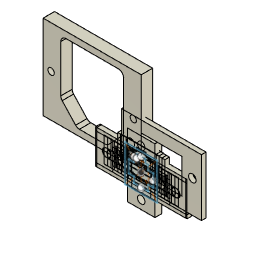
Panel Mount Profiles (Autodesk Fusion 360 design; units mm, degrees)
Autodesk Fusion 360 part; units mm, degrees
(part 1 of 2)
sketch "MF3 1R 2P" plane through (0, 0, 0) normal (0, 1, 0) x (1, 0, 0) in component "Molex Micro Fit 3"
  line L0 (5.75, 1.575) -> (-5.75, 1.575) construction
  line L1 (-5.75, 1.575) -> (-5.75, -1.575)
  line L2 (-5.75, -1.575) -> (5.75, -1.575) construction
  line L3 (5.75, -1.575) -> (5.75, 1.575)
  line L4 (5.75, 1.575) -> (-5.75, -1.575) construction
  line L5 (-5.75, 1.575) -> (5.75, -1.575) construction
  line L6 (3.575, 2.075) -> (-3.575, 2.075)
  line L7 (-3.575, 2.075) -> (-3.575, -2.075) construction
  line L8 (-3.575, -2.075) -> (3.575, -2.075) construction
  line L9 (3.575, -2.075) -> (3.575, 2.075) construction
  line L10 (3.575, 2.075) -> (-3.575, -2.075) construction
  line L11 (-3.575, 2.075) -> (3.575, -2.075) construction
  line L12 (0, -2.075) -> (0, -3.275) construction
  line L13 (1.45, -3.275) -> (-1.45, -3.275)
  line L14 (-1.45, -3.275) -> (-1.45, -2.075)
  line L15 (-1.45, -2.075) -> (1.45, -2.075) construction
  line L16 (1.45, -2.075) -> (1.45, -3.275)
  line L17 (1.45, -3.275) -> (-1.45, -2.075) construction
  line L18 (-1.45, -3.275) -> (1.45, -2.075) construction
  line L19 (3.575, 1.575) -> (3.575, 2.075)
  line L20 (3.575, 1.575) -> (5.75, 1.575)
  line L21 (-5.75, 1.575) -> (-3.575, 1.575)
  line L22 (-3.575, 1.575) -> (-3.575, 2.075)
  line L23 (-5.75, -1.575) -> (-3.575, -1.575)
  line L24 (-3.575, -1.575) -> (-3.575, -2.075)
  line L25 (-3.575, -2.075) -> (-1.45, -2.075)
  line L26 (1.45, -2.075) -> (3.575, -2.075)
  line L27 (3.575, -2.075) -> (3.575, -1.575)
  line L28 (3.575, -1.575) -> (5.75, -1.575)
  line L29 (0, -3.275) -> (0, 2.075) construction
  line L30 (7.25, 3.4) -> (-7.25, 3.4)
  line L31 (-7.25, 3.4) -> (-7.25, -4.6)
  line L32 (-7.25, -4.6) -> (7.25, -4.6)
  line L33 (7.25, -4.6) -> (7.25, 3.4)
  line L34 (7.25, 3.4) -> (-7.25, -4.6) construction
  line L35 (-7.25, 3.4) -> (7.25, -4.6) construction
  point P0 (0, -2.675)
  point P1 (0, -0.6)
  dimension "d223" = 11.5
  dimension "d224" = 3.15
  dimension "d225" = 7.15
  dimension "d226" = 4.15
  dimension "d227" = 1.2
  dimension "d228" = 2.9
  dimension "d229" = 14.5
  dimension "d230" = 5.35
  dimension "d231" = 8
  constraint horizontal L0
  constraint perpendicular L0 L1
  constraint parallel L0 L2
  constraint parallel L1 L3
  constraint coincident L4 origin
  constraint coincident L5 origin
  constraint horizontal L6
  constraint perpendicular L6 L7
  constraint parallel L6 L8
  constraint parallel L7 L9
  constraint coincident L10 origin
  constraint coincident L11 origin
  constraint midpoint L8 L12.start
  constraint perpendicular L8 L12
  constraint horizontal L13
  constraint perpendicular L13 L14
  constraint parallel L13 L15
  constraint parallel L14 L16
  constraint coincident L17 P0
  constraint coincident L18 P0
  constraint midpoint L12 P0
  constraint coincident L0 L19.start
  constraint coincident L9 L19.start
  constraint perpendicular L3 L20
  constraint coincident L0 L21.end
  constraint coincident L7 L21.end
  constraint coincident L2 L23.end
  constraint coincident L7 L23.end
  constraint perpendicular L14 L25
  constraint coincident L2 L27.end
  constraint coincident L9 L27.end
  constraint midpoint L6 L29.end
  constraint horizontal L30
  constraint perpendicular L30 L31
  constraint parallel L30 L32
  constraint parallel L31 L33
  constraint coincident L34 P1
  constraint coincident L35 P1
  constraint midpoint L29 P1
  measures "d223" distance of L1.end L2.end
  measures "d224" distance of L0.end L1.end
  measures "d225" distance of L7.end L8.end
  measures "d226" distance of L6.end L7.end
  measures "d227" distance of L12.start L12.end
  measures "d228" distance of L14.end L15.end
  measures "d229" distance of L31.end L32.end
  measures "d230" distance of L6 L13
  measures "d231" distance of L30.end L31.end
sketch "MF3 2R 2P" plane through (0, 0, 0) normal (0, 1, 0) x (1, 0, 0) in component "Molex Micro Fit 3"
  line L0 (-5.6125, 4.8465) -> (5.8875, 4.8465)
  line L1 (5.8875, 4.8465) -> (5.8875, -6.1535)
  line L2 (5.8875, -6.1535) -> (-5.6125, -6.1535)
  line L3 (-5.6125, -6.1535) -> (-5.6125, 4.8465)
  line L4 (-5.6125, 4.8465) -> (5.8875, -6.1535) construction
  line L5 (5.8875, 4.8465) -> (-5.6125, -6.1535) construction
  line L6 (4.25, 1.875) -> (-4.25, 1.875) construction
  line L7 (-4.25, 1.875) -> (-4.25, -1.875)
  line L8 (-4.25, -1.875) -> (4.25, -1.875) construction
  line L9 (4.25, -1.875) -> (4.25, 1.875)
  line L10 (4.25, 1.875) -> (-4.25, -1.875) construction
  line L11 (-4.25, 1.875) -> (4.25, -1.875) construction
  line L12 (2.075, 3.575) -> (-2.075, 3.575)
  line L13 (-2.075, 3.575) -> (-2.075, -3.575) construction
  line L14 (-2.075, -3.575) -> (2.075, -3.575) construction
  line L15 (2.075, -3.575) -> (2.075, 3.575) construction
  line L16 (2.075, 3.575) -> (-2.075, -3.575) construction
  line L17 (-2.075, 3.575) -> (2.075, -3.575) construction
  line L18 (0, -3.575) -> (0, -4.775) construction
  line L19 (0.85, -4.775) -> (-0.85, -4.775)
  line L20 (-0.85, -4.775) -> (-0.85, -3.575)
  line L21 (-0.85, -3.575) -> (0.85, -3.575) construction
  line L22 (0.85, -3.575) -> (0.85, -4.775)
  line L23 (0.85, -4.775) -> (-0.85, -3.575) construction
  line L24 (-0.85, -4.775) -> (0.85, -3.575) construction
  line L25 (0.1375, -6.1535) -> (0.1375, 4.8465) construction
  line L26 (0.85, -3.575) -> (2.075, -3.575)
  line L27 (2.075, -1.875) -> (4.25, -1.875)
  line L28 (2.075, -1.875) -> (2.075, -3.575)
  line L29 (4.25, 1.875) -> (2.075, 1.875)
  line L30 (2.075, 1.875) -> (2.075, 3.575)
  line L31 (-2.075, 3.575) -> (-2.075, 1.875)
  line L32 (-2.075, 1.875) -> (-4.25, 1.875)
  line L33 (-4.25, -1.875) -> (-2.075, -1.875)
  line L34 (-2.075, -1.875) -> (-2.075, -3.575)
  line L35 (-2.075, -3.575) -> (-0.85, -3.575)
  point P0 (0.1375, -0.6535)
  point P1 (0, -4.175)
  dimension "d105" = 11.5
  dimension "d106" = 11
  dimension "d162" = 8.5
  dimension "d163" = 3.75
  dimension "d164" = 4.15
  dimension "d165" = 7.15
  dimension "d166" = 1.2
  dimension "d167" = 1.7
  constraint horizontal L0
  constraint perpendicular L0 L1
  constraint parallel L0 L2
  constraint parallel L1 L3
  constraint coincident L4 P0
  constraint coincident L5 P0
  constraint horizontal L6
  constraint perpendicular L6 L7
  constraint parallel L6 L8
  constraint parallel L7 L9
  constraint coincident L10 origin
  constraint coincident L11 origin
  constraint horizontal L12
  constraint perpendicular L12 L13
  constraint parallel L12 L14
  constraint parallel L13 L15
  constraint coincident L16 origin
  constraint coincident L17 origin
  constraint midpoint L14 L18.start
  constraint perpendicular L14 L18
  constraint horizontal L19
  constraint perpendicular L19 L20
  constraint parallel L19 L21
  constraint parallel L20 L22
  constraint coincident L23 P1
  constraint coincident L24 P1
  constraint midpoint L18 P1
  constraint coincident L18.end L19
  constraint midpoint L2 L25.start
  constraint midpoint L0 L25.end
  constraint coincident L15 L27.start
  constraint coincident L8 L27.start
  constraint coincident L6 L29.end
  constraint coincident L15 L29.end
  constraint coincident L13 L31.end
  constraint coincident L6 L31.end
  constraint coincident L13 L33.end
  constraint coincident L8 L33.end
  measures "d105" distance of L1.end L2.end
  measures "d106" distance of L0.end L1.end
  measures "d162" distance of L7.end L8.end
  measures "d163" distance of L6.end L7.end
  measures "d164" distance of L13.end L14.end
  measures "d165" distance of L12.end L13.end
  measures "d166" distance of L18.start L18.end
  measures "d167" distance of L20.end L21.end
sketch "MF3 1R 3P" plane through (0, 0, 0) normal (0, 1, 0) x (1, 0, 0) in component "Molex Micro Fit 3"
  line L0 (0.0006, -3.28) -> (0.0006, 2.09) construction
  line L1 (5.0756, -2.06) -> (5.0756, 2.09) construction
  line L2 (5.0756, 2.09) -> (-5.0744, 2.09)
  line L3 (-5.0744, 2.09) -> (-5.0744, -2.08) construction
  line L4 (-5.0744, -2.08) -> (-1.4494, -2.08)
  line L5 (-1.4494, -3.28) -> (-1.4494, -2.08)
  line L6 (1.4506, -3.28) -> (-1.4494, -3.28)
  line L7 (1.4506, -2.06) -> (1.4506, -3.28)
  line L8 (1.4506, -2.06) -> (5.0756, -2.06)
  line L9 (7.25, -1.575) -> (-7.25, -1.575) construction
  line L10 (-7.25, -1.575) -> (-7.25, 1.575)
  line L11 (-7.25, 1.575) -> (7.25, 1.575) construction
  line L12 (7.25, 1.575) -> (7.25, -1.575)
  line L13 (7.25, -1.575) -> (-7.25, 1.575) construction
  line L14 (-7.25, -1.575) -> (7.25, 1.575) construction
  line L15 (-5.0744, -2.08) -> (-5.0744, -1.575)
  line L16 (-5.0744, -1.575) -> (-7.25, -1.575)
  line L17 (-7.25, 1.575) -> (-5.0744, 1.575)
  line L18 (-5.0744, 1.575) -> (-5.0744, 2.09)
  line L19 (5.0756, 2.09) -> (5.0756, 1.5652)
  line L20 (5.0756, 1.5652) -> (7.25, 1.575)
  line L21 (7.25, -1.575) -> (5.0756, -1.575)
  line L22 (5.0756, -1.575) -> (5.0756, -2.06)
  line L23 (8.7506, 3.405) -> (-8.7494, 3.405)
  line L24 (-8.7494, 3.405) -> (-8.7494, -4.595)
  line L25 (-8.7494, -4.595) -> (8.7506, -4.595)
  line L26 (8.7506, -4.595) -> (8.7506, 3.405)
  line L27 (8.7506, 3.405) -> (-8.7494, -4.595) construction
  line L28 (-8.7494, 3.405) -> (8.7506, -4.595) construction
  point P0 (0.0006, -0.595)
  dimension "d96" = 14.5
  dimension "d97" = 3.15
  dimension "d98" = 17.5
  dimension "d99" = 8
  dimension "d129" = 1.2
  dimension "d130" = 2.9
  dimension "d131" = 4.15
  dimension "d132" = 10.15
  dimension "d133" = 5.37
  constraint horizontal L9
  constraint perpendicular L9 L10
  constraint parallel L9 L11
  constraint parallel L10 L12
  constraint coincident L13 origin
  constraint coincident L14 origin
  constraint coincident L9 L15.end
  constraint coincident L3 L15.end
  constraint coincident L11 L17.end
  constraint coincident L3 L17.end
  constraint coincident L1 L19.end
  constraint coincident L9 L21.end
  constraint coincident L1 L21.end
  constraint horizontal L23
  constraint perpendicular L23 L24
  constraint parallel L23 L25
  constraint parallel L24 L26
  constraint coincident L27 P0
  constraint coincident L28 P0
  constraint midpoint L0 P0
  constraint midpoint L0.start L6
  constraint midpoint L0.end L2
  constraint horizontal L8
  constraint horizontal L4
  constraint horizontal L2
  constraint vertical L3
  constraint vertical L1
  constraint vertical L5
  constraint vertical L7
  constraint symmetric L0 L24 L26
  measures "d96" distance of L10.end L11.end
  measures "d97" distance of L9.end L10.end
  measures "d98" distance of L24.end L25.end
  measures "d99" distance of L23.end L24.end
  measures "d129" distance of L4.end L5.start
  measures "d130" distance of L5.start L6.start
  measures "d131" distance of L1.start L1.end
  measures "d132" distance of L1.end L2.end
  measures "d133" distance of L2 L6
sketch "MF3 1R 4P" plane through (0, 0, 0) normal (0, 1, 0) x (1, 0, 0) in component "Molex Micro Fit 3"
  line L0 (6.575, 2.075) -> (-6.575, 2.075)
  line L1 (6.575, 2.075) -> (-6.575, -2.075) construction
  line L2 (-6.575, 2.075) -> (6.575, -2.075) construction
  line L3 (0, -2.075) -> (0, -3.275) construction
  line L4 (1.45, -3.275) -> (-1.45, -3.275)
  line L5 (-1.45, -3.275) -> (-1.45, -2.075)
  line L6 (-1.45, -2.075) -> (1.45, -2.075) construction
  line L7 (1.45, -2.075) -> (1.45, -3.275)
  line L8 (1.45, -3.275) -> (-1.45, -2.075) construction
  line L9 (-1.45, -3.275) -> (1.45, -2.075) construction
  line L10 (-6.575, -2.075) -> (-1.45, -2.075)
  line L11 (0, -2.075) -> (6.575, -2.075)
  line L12 (8.75, 1.575) -> (-8.75, 1.575)
  line L13 (-8.75, 1.575) -> (-8.75, -1.575)
  line L14 (-8.75, -1.575) -> (8.75, -1.575)
  line L15 (8.75, -1.575) -> (8.75, 1.575)
  line L16 (8.75, 1.575) -> (-8.75, -1.575) construction
  line L17 (-8.75, 1.575) -> (8.75, -1.575) construction
  line L18 (6.575, -2.075) -> (6.575, -1.575)
  line L19 (6.575, 1.575) -> (6.575, 2.075)
  line L20 (-6.575, 2.075) -> (-6.575, 1.575)
  line L21 (-6.575, -1.575) -> (-6.575, -2.075)
  line L22 (0, -3.275) -> (0, 2.075) construction
  line L23 (10.75, 3.4) -> (-10.75, 3.4)
  line L24 (-10.75, 3.4) -> (-10.75, -4.6)
  line L25 (-10.75, -4.6) -> (10.75, -4.6)
  line L26 (10.75, -4.6) -> (10.75, 3.4)
  line L27 (10.75, 3.4) -> (-10.75, -4.6) construction
  line L28 (-10.75, 3.4) -> (10.75, -4.6) construction
  point P0 (0, -2.675)
  point P1 (0, -0.6)
  dimension "d120" = 13.15
  dimension "d121" = 4.15
  dimension "d122" = 1.2
  dimension "d123" = 2.9
  dimension "d124" = 17.5
  dimension "d125" = 3.15
  dimension "d126" = 5.35
  dimension "d127" = 8
  dimension "d128" = 21.5
  constraint horizontal L0
  constraint perpendicular L0 L20
  constraint parallel L0 L10
  constraint parallel L18 L20
  constraint coincident L1 origin
  constraint coincident L2 origin
  constraint perpendicular L3 L10
  constraint horizontal L4
  constraint perpendicular L4 L5
  constraint parallel L4 L6
  constraint parallel L5 L7
  constraint coincident L8 P0
  constraint coincident L9 P0
  constraint midpoint L3 P0
  constraint collinear L10 L11
  constraint coincident L3.start L10
  constraint horizontal L12
  constraint perpendicular L12 L13
  constraint parallel L12 L14
  constraint parallel L13 L15
  constraint coincident L16 origin
  constraint coincident L17 origin
  constraint collinear L18 L19
  constraint collinear L20 L21
  constraint coincident L14 L21.start
  constraint coincident L12 L20.end
  constraint coincident L12 L19.start
  constraint coincident L14 L18.end
  constraint midpoint L0 L22.end
  constraint perpendicular L0 L22
  constraint horizontal L23
  constraint perpendicular L23 L24
  constraint parallel L23 L25
  constraint parallel L24 L26
  constraint coincident L27 P1
  constraint coincident L28 P1
  constraint midpoint L22 P1
  measures "d120" distance of L1.end L2.end
  measures "d121" distance of L0.end L1.end
  measures "d122" distance of L3.start L3.end
  measures "d123" distance of L5.end L6.end
  measures "d124" distance of L13.end L14.end
  measures "d125" distance of L12.end L13.end
  measures "d126" distance of L0 L4
  measures "d127" distance of L23.end L24.end
  measures "d128" distance of L23.start L23.end
sketch "MF3 1R 5P" plane through (0, 0, 0) normal (0, 1, 0) x (1, 0, 0) in component "Molex Micro Fit 3"
  line L0 (10.25, 1.575) -> (-10.25, 1.575)
  line L1 (-10.25, 1.575) -> (-10.25, -1.575)
  line L2 (-10.25, -1.575) -> (10.25, -1.575)
  line L3 (10.25, -1.575) -> (10.25, 1.575)
  line L4 (10.25, 1.575) -> (-10.25, -1.575) construction
  line L5 (-10.25, 1.575) -> (10.25, -1.575) construction
  line L6 (8.075, 2.075) -> (-8.075, 2.075)
  line L7 (-8.075, 2.075) -> (-8.075, -2.075)
  line L8 (-8.075, -2.075) -> (8.075, -2.075)
  line L9 (8.075, -2.075) -> (8.075, 2.075)
  line L10 (8.075, 2.075) -> (-8.075, -2.075) construction
  line L11 (-8.075, 2.075) -> (8.075, -2.075) construction
  line L12 (0, -2.075) -> (0, -3.275) construction
  line L13 (1.45, -2.075) -> (-1.45, -2.075)
  line L14 (-1.45, -2.075) -> (-1.45, -3.275)
  line L15 (-1.45, -3.275) -> (1.45, -3.275)
  line L16 (1.45, -3.275) -> (1.45, -2.075)
  line L17 (1.45, -2.075) -> (-1.45, -3.275) construction
  line L18 (-1.45, -2.075) -> (1.45, -3.275) construction
  line L19 (0, -3.275) -> (0, 2.075) construction
  line L20 (11.25, 3.4) -> (-11.25, 3.4)
  line L21 (-11.25, 3.4) -> (-11.25, -4.6)
  line L22 (-11.25, -4.6) -> (11.25, -4.6)
  line L23 (11.25, -4.6) -> (11.25, 3.4)
  line L24 (11.25, 3.4) -> (-11.25, -4.6) construction
  line L25 (-11.25, 3.4) -> (11.25, -4.6) construction
  point P0 (0, -2.675)
  point P1 (0, -0.6)
  dimension "d134" = 20.5
  dimension "d135" = 3.15
  dimension "d136" = 16.15
  dimension "d137" = 4.15
  dimension "d138" = 1.2
  dimension "d139" = 2.9
  dimension "d140" = 1.2
  dimension "d141" = 5.35
  dimension "d142" = 22.5
  dimension "d143" = 8
  constraint horizontal L0
  constraint perpendicular L0 L1
  constraint parallel L0 L2
  constraint parallel L1 L3
  constraint coincident L4 origin
  constraint coincident L5 origin
  constraint horizontal L6
  constraint perpendicular L6 L7
  constraint parallel L6 L8
  constraint parallel L7 L9
  constraint coincident L10 origin
  constraint coincident L11 origin
  constraint midpoint L8 L12.start
  constraint perpendicular L8 L12
  constraint horizontal L13
  constraint perpendicular L13 L14
  constraint parallel L13 L15
  constraint parallel L14 L16
  constraint coincident L17 P0
  constraint coincident L18 P0
  constraint midpoint L12 P0
  constraint midpoint L6 L19.end
  constraint horizontal L20
  constraint perpendicular L20 L21
  constraint parallel L20 L22
  constraint parallel L21 L23
  constraint coincident L24 P1
  constraint coincident L25 P1
  constraint midpoint L19 P1
  measures "d134" distance of L1.end L2.end
  measures "d135" distance of L0.end L1.end
  measures "d136" distance of L7.end L8.end
  measures "d137" distance of L6.end L7.end
  measures "d138" distance of L12.start L12.end
  measures "d139" distance of L14.end L15.end
  measures "d140" distance of L13.end L14.end
  measures "d141" distance of L6 L15
  measures "d142" distance of L21.end L22.end
  measures "d143" distance of L20.end L21.end
sketch "MF3 2R 4P" plane through (0, 0, 0) normal (0, 1, 0) x (1, 0, 0) in component "Molex Micro Fit 3"
  line L0 (3.575, 3.45) -> (-3.575, 3.45)
  line L1 (-3.575, 3.45) -> (-3.575, -3.45) construction
  line L2 (-3.575, -3.45) -> (3.575, -3.45) construction
  line L3 (3.575, -3.45) -> (3.575, 3.45) construction
  line L4 (3.575, 3.45) -> (-3.575, -3.45) construction
  line L5 (-3.575, 3.45) -> (3.575, -3.45) construction
  line L6 (5.75, 1.875) -> (-5.75, 1.875) construction
  line L7 (-5.75, 1.875) -> (-5.75, -1.875)
  line L8 (-5.75, -1.875) -> (5.75, -1.875) construction
  line L9 (5.75, -1.875) -> (5.75, 1.875)
  line L10 (5.75, 1.875) -> (-5.75, -1.875) construction
  line L11 (-5.75, 1.875) -> (5.75, -1.875) construction
  line L12 (0, -3.45) -> (0, -4.85) construction
  line L13 (0.85, -4.85) -> (-0.85, -4.85)
  line L14 (-0.85, -4.85) -> (-0.85, -3.45)
  line L15 (0.85, -3.45) -> (0.85, -4.85)
  line L16 (0.85, -4.85) -> (-0.85, -3.45) construction
  line L17 (-0.85, -4.85) -> (0.85, -3.45) construction
  line L18 (5.75, -1.875) -> (3.575, -1.875)
  line L19 (3.575, -1.875) -> (3.575, -3.45)
  line L20 (3.575, -3.45) -> (0.85, -3.45)
  line L21 (-0.85, -3.45) -> (-3.575, -3.45)
  line L22 (-3.575, -3.45) -> (-3.575, -1.875)
  line L23 (-3.575, -1.875) -> (-5.75, -1.875)
  line L24 (-5.75, 1.875) -> (-3.575, 1.875)
  line L25 (-3.575, 1.875) -> (-3.575, 3.45)
  line L26 (3.575, 3.45) -> (3.575, 1.875)
  line L27 (3.575, 1.875) -> (5.75, 1.875)
  line L28 (0, -4.85) -> (0, 3.45) construction
  line L29 (7.25, 4.8) -> (-7.25, 4.8)
  line L30 (-7.25, 4.8) -> (-7.25, -6.2)
  line L31 (-7.25, -6.2) -> (7.25, -6.2)
  line L32 (7.25, -6.2) -> (7.25, 4.8)
  line L33 (7.25, 4.8) -> (-7.25, -6.2) construction
  line L34 (-7.25, 4.8) -> (7.25, -6.2) construction
  point P0 (0, -4.15)
  point P1 (0, -0.7)
  point P2 (0, -0.7)
  dimension "d176" = 7.15
  dimension "d177" = 6.9
  dimension "d178" = 11.5
  dimension "d179" = 3.75
  dimension "d180" = 1.4
  dimension "d181" = 1.7
  dimension "d184" = 11
  dimension "d185" = 14.5
  constraint horizontal L0
  constraint perpendicular L0 L1
  constraint parallel L0 L2
  constraint parallel L1 L3
  constraint coincident L4 origin
  constraint coincident L5 origin
  constraint horizontal L6
  constraint perpendicular L6 L7
  constraint parallel L6 L8
  constraint parallel L7 L9
  constraint coincident L10 origin
  constraint coincident L11 origin
  constraint midpoint L2 L12.start
  constraint perpendicular L2 L12
  constraint horizontal L13
  constraint perpendicular L13 L14
  constraint parallel L14 L15
  constraint coincident L16 P0
  constraint coincident L17 P0
  constraint midpoint L12 P0
  constraint coincident L12.end L13
  constraint coincident L8 L18.end
  constraint coincident L3 L18.end
  constraint perpendicular L15 L20
  constraint coincident L1 L22.end
  constraint coincident L8 L22.end
  constraint coincident L1 L24.end
  constraint coincident L6 L24.end
  constraint coincident L3 L26.end
  constraint coincident L6 L26.end
  constraint midpoint L0 L28.end
  constraint midpoint L28 P2
  constraint horizontal L29
  constraint perpendicular L29 L30
  constraint parallel L29 L31
  constraint parallel L30 L32
  constraint coincident L33 P2
  constraint coincident L34 P2
  constraint coincident P2 P1
  measures "d176" distance of L1.end L2.end
  measures "d177" distance of L0.end L1.end
  measures "d178" distance of L7.end L8.end
  measures "d179" distance of L6.end L7.end
  measures "d180" distance of L12.start L12.end
  measures "d181" distance of L14.end L15.start
  measures "d184" distance of L29.end L30.end
  measures "d185" distance of L30 L32
sketch "MF3 2R 8P" plane through (0, 0, 0) normal (0, 1, 0) x (1, 0, 0) in component "Molex Micro Fit 3"
  line L0 (6.575, 3.575) -> (-6.575, 3.575)
  line L1 (-6.575, 3.575) -> (-6.575, -3.575) construction
  line L2 (-6.575, -3.575) -> (6.575, -3.575) construction
  line L3 (6.575, -3.575) -> (6.575, 3.575) construction
  line L4 (6.575, 3.575) -> (-6.575, -3.575) construction
  line L5 (-6.575, 3.575) -> (6.575, -3.575) construction
  line L6 (8.75, 1.875) -> (-8.75, 1.875) construction
  line L7 (-8.75, 1.875) -> (-8.75, -1.875)
  line L8 (-8.75, -1.875) -> (8.75, -1.875) construction
  line L9 (8.75, -1.875) -> (8.75, 1.875)
  line L10 (8.75, 1.875) -> (-8.75, -1.875) construction
  line L11 (-8.75, 1.875) -> (8.75, -1.875) construction
  line L12 (0, -3.575) -> (0, -4.975) construction
  line L13 (0.85, -3.575) -> (-0.85, -3.575) construction
  line L14 (-0.85, -3.575) -> (-0.85, -4.975)
  line L15 (-0.85, -4.975) -> (0.85, -4.975)
  line L16 (0.85, -4.975) -> (0.85, -3.575)
  line L17 (0.85, -3.575) -> (-0.85, -4.975) construction
  line L18 (-0.85, -3.575) -> (0.85, -4.975) construction
  line L19 (8.75, -1.875) -> (6.575, -1.875)
  line L20 (6.575, -1.875) -> (6.575, -3.575)
  line L21 (6.575, -3.575) -> (0.85, -3.575)
  line L22 (8.75, 1.875) -> (6.575, 1.875)
  line L23 (6.575, 1.875) -> (6.575, 3.575)
  line L24 (-6.575, 3.575) -> (-6.575, 1.875)
  line L25 (-6.575, 1.875) -> (-8.75, 1.875)
  line L26 (-8.75, -1.875) -> (-6.575, -1.875)
  line L27 (-6.575, -1.875) -> (-6.575, -3.575)
  line L28 (-6.575, -3.575) -> (-0.85, -3.575)
  line L29 (0, -4.975) -> (0, 3.575) construction
  line L30 (10.25, 4.8) -> (-10.25, 4.8)
  line L31 (-10.25, 4.8) -> (-10.25, -6.2)
  line L32 (-10.25, -6.2) -> (10.25, -6.2)
  line L33 (10.25, -6.2) -> (10.25, 4.8)
  line L34 (10.25, 4.8) -> (-10.25, -6.2) construction
  line L35 (-10.25, 4.8) -> (10.25, -6.2) construction
  point P0 (0, -4.275)
  point P1 (0, -0.7)
  dimension "d186" = 13.15
  dimension "d187" = 7.15
  dimension "d188" = 17.5
  dimension "d189" = 3.75
  dimension "d190" = 1.4
  dimension "d191" = 1.7
  dimension "d192" = 20.5
  dimension "d193" = 11
  constraint horizontal L0
  constraint perpendicular L0 L1
  constraint parallel L0 L2
  constraint parallel L1 L3
  constraint coincident L4 origin
  constraint coincident L5 origin
  constraint horizontal L6
  constraint perpendicular L6 L7
  constraint parallel L6 L8
  constraint parallel L7 L9
  constraint coincident L10 origin
  constraint coincident L11 origin
  constraint midpoint L2 L12.start
  constraint perpendicular L2 L12
  constraint horizontal L13
  constraint perpendicular L13 L14
  constraint parallel L13 L15
  constraint parallel L14 L16
  constraint coincident L17 P0
  constraint coincident L18 P0
  constraint midpoint L12 P0
  constraint coincident L12.end L15
  constraint coincident L8 L19.end
  constraint coincident L3 L19.end
  constraint coincident L6 L22.end
  constraint coincident L3 L22.end
  constraint coincident L6 L24.end
  constraint coincident L1 L24.end
  constraint coincident L8 L26.end
  constraint coincident L1 L26.end
  constraint midpoint L0 L29.end
  constraint horizontal L30
  constraint perpendicular L30 L31
  constraint parallel L30 L32
  constraint parallel L31 L33
  constraint coincident L34 P1
  constraint coincident L35 P1
  constraint midpoint L29 P1
  measures "d186" distance of L1.end L2.end
  measures "d187" distance of L0.end L1.end
  measures "d188" distance of L7.end L8.end
  measures "d189" distance of L6.end L7.end
  measures "d190" distance of L12.start L12.end
  measures "d191" distance of L14.end L15.end
  measures "d192" distance of L31.end L32.end
  measures "d193" distance of L30.end L31.end
sketch "MF3 2R 6P" plane through (0, 0, 0) normal (0, 1, 0) x (1, 0, 0) in component "Molex Micro Fit 3"
  line L0 (5.075, 3.575) -> (-5.075, 3.575)
  line L1 (-5.075, 3.575) -> (-5.075, -3.575) construction
  line L2 (-5.075, -3.575) -> (5.075, -3.575) construction
  line L3 (5.075, -3.575) -> (5.075, 3.575) construction
  line L4 (5.075, 3.575) -> (-5.075, -3.575) construction
  line L5 (-5.075, 3.575) -> (5.075, -3.575) construction
  line L6 (7.25, 1.875) -> (-7.25, 1.875) construction
  line L7 (-7.25, 1.875) -> (-7.25, -1.875)
  line L8 (-7.25, -1.875) -> (7.25, -1.875) construction
  line L9 (7.25, -1.875) -> (7.25, 1.875)
  line L10 (7.25, 1.875) -> (-7.25, -1.875) construction
  line L11 (-7.25, 1.875) -> (7.25, -1.875) construction
  line L12 (0, -3.575) -> (0, -4.975) construction
  line L13 (0.85, -4.975) -> (-0.85, -4.975)
  line L14 (-0.85, -4.975) -> (-0.85, -3.575)
  line L15 (-0.85, -3.575) -> (0.85, -3.575) construction
  line L16 (0.85, -3.575) -> (0.85, -4.975)
  line L17 (0.85, -4.975) -> (-0.85, -3.575) construction
  line L18 (-0.85, -4.975) -> (0.85, -3.575) construction
  line L19 (-0.85, -3.575) -> (-5.075, -3.575)
  line L20 (-5.075, -3.575) -> (-5.075, -1.875)
  line L21 (-5.075, -1.875) -> (-7.25, -1.875)
  line L22 (-7.25, 1.875) -> (-5.075, 1.875)
  line L23 (-5.075, 1.875) -> (-5.075, 3.575)
  line L24 (5.075, 1.875) -> (5.075, 3.575)
  line L25 (5.075, 1.875) -> (7.25, 1.875)
  line L26 (5.075, -3.575) -> (5.075, -1.875)
  line L27 (5.075, -1.875) -> (7.25, -1.875)
  line L28 (0.85, -3.575) -> (5.075, -3.575)
  line L29 (0, -4.975) -> (0, 3.575) construction
  line L30 (8.75, -6.2) -> (-8.75, -6.2)
  line L31 (-8.75, -6.2) -> (-8.75, 4.8)
  line L32 (-8.75, 4.8) -> (8.75, 4.8)
  line L33 (8.75, 4.8) -> (8.75, -6.2)
  line L34 (8.75, -6.2) -> (-8.75, 4.8) construction
  line L35 (-8.75, -6.2) -> (8.75, 4.8) construction
  point P0 (0, -4.275)
  point P1 (0, -0.7)
  dimension "d305" = 10.15
  dimension "d306" = 7.15
  dimension "d307" = 14.5
  dimension "d308" = 3.75
  dimension "d309" = 1.4
  dimension "d310" = 1.7
  dimension "d312" = 17.5
  dimension "d313" = 11
  constraint horizontal L0
  constraint perpendicular L0 L1
  constraint parallel L0 L2
  constraint parallel L1 L3
  constraint coincident L4 origin
  constraint coincident L5 origin
  constraint horizontal L6
  constraint perpendicular L6 L7
  constraint parallel L6 L8
  constraint parallel L7 L9
  constraint coincident L10 origin
  constraint coincident L11 origin
  constraint midpoint L2 L12.start
  constraint perpendicular L2 L12
  constraint horizontal L13
  constraint perpendicular L13 L14
  constraint parallel L13 L15
  constraint parallel L14 L16
  constraint coincident L17 P0
  constraint coincident L18 P0
  constraint midpoint L12 P0
  constraint perpendicular L1 L19
  constraint coincident L8 L20.end
  constraint coincident L1 L20.end
  constraint coincident L6 L22.end
  constraint coincident L1 L22.end
  constraint coincident L6 L24.start
  constraint coincident L3 L24.start
  constraint coincident L3 L26.end
  constraint coincident L8 L26.end
  constraint midpoint L0 L29.end
  constraint horizontal L30
  constraint perpendicular L30 L31
  constraint parallel L30 L32
  constraint parallel L31 L33
  constraint coincident L34 P1
  constraint coincident L35 P1
  constraint midpoint L29 P1
  measures "d305" distance of L1.end L2.end
  measures "d306" distance of L0.end L1.end
  measures "d307" distance of L7.end L8.end
  measures "d308" distance of L6.end L7.end
  measures "d309" distance of L12.start L12.end
  measures "d310" distance of L14.end L15.end
  measures "d312" distance of L30.start L30.end
  measures "d313" distance of L30.end L31.end
sketch "MF3 2R 10P" plane through (0, 0, 0) normal (0, 1, 0) x (1, 0, 0) in component "Molex Micro Fit 3"
  line L0 (11.75, -6.2) -> (-11.75, -6.2)
  line L1 (-8.075, -3.575) -> (8.075, -3.575) construction
  line L2 (0.85, -4.975) -> (-0.85, -4.975)
  line L3 (11.75, 4.8) -> (11.75, -6.2)
  line L4 (-11.75, 4.8) -> (11.75, 4.8)
  line L5 (-10.25, 1.875) -> (-8.075, 1.875)
  line L6 (0, -4.975) -> (0, 3.575) construction
  line L7 (10.25, 1.875) -> (-10.25, 1.875) construction
  line L8 (0, -3.575) -> (0, -4.975) construction
  line L9 (0.85, -3.575) -> (8.075, -3.575)
  line L10 (0.85, -4.975) -> (-0.85, -3.575) construction
  line L11 (8.075, 1.875) -> (8.075, 3.575)
  line L12 (8.075, 1.875) -> (10.25, 1.875)
  line L13 (0.85, -3.575) -> (0.85, -4.975)
  line L14 (-10.25, -1.875) -> (10.25, -1.875) construction
  line L15 (-8.075, -3.575) -> (-8.075, -1.875)
  line L16 (10.25, -1.875) -> (10.25, 1.875)
  line L17 (-8.075, 3.575) -> (-8.075, -3.575) construction
  line L18 (11.75, -6.2) -> (-11.75, 4.8) construction
  line L19 (-0.85, -3.575) -> (-8.075, -3.575)
  line L20 (-0.85, -4.975) -> (-0.85, -3.575)
  line L21 (-0.85, -4.975) -> (0.85, -3.575) construction
  line L22 (8.075, -1.875) -> (10.25, -1.875)
  line L23 (8.075, -3.575) -> (8.075, 3.575) construction
  line L24 (-11.75, -6.2) -> (11.75, 4.8) construction
  line L25 (-10.25, 1.875) -> (10.25, -1.875) construction
  line L26 (10.25, 1.875) -> (-10.25, -1.875) construction
  line L27 (8.075, 3.575) -> (-8.075, -3.575) construction
  line L28 (8.075, 3.575) -> (-8.075, 3.575)
  line L29 (-10.25, 1.875) -> (-10.25, -1.875)
  line L30 (-0.85, -3.575) -> (0.85, -3.575) construction
  line L31 (-8.075, 3.575) -> (8.075, -3.575) construction
  line L32 (-11.75, -6.2) -> (-11.75, 4.8)
  line L33 (-8.075, -1.875) -> (-10.25, -1.875)
  line L34 (-8.075, 1.875) -> (-8.075, 3.575)
  line L35 (8.075, -3.575) -> (8.075, -1.875)
  point P0 (0, -0.7)
  point P1 (0, -4.275)
  dimension "d314" = 16.15
  dimension "d315" = 7.15
  dimension "d316" = 20.5
  dimension "d317" = 3.75
  dimension "d318" = 1.4
  dimension "d319" = 1.7
  dimension "d320" = 23.5
  dimension "d321" = 11
  constraint horizontal L28
  constraint perpendicular L17 L28
  constraint parallel L1 L28
  constraint parallel L17 L23
  constraint coincident origin L27
  constraint coincident origin L31
  constraint horizontal L7
  constraint perpendicular L7 L29
  constraint parallel L7 L14
  constraint parallel L16 L29
  constraint coincident origin L26
  constraint coincident origin L25
  constraint midpoint L8.start L1
  constraint perpendicular L1 L8
  constraint horizontal L2
  constraint perpendicular L2 L20
  constraint parallel L2 L30
  constraint parallel L13 L20
  constraint coincident P1 L10
  constraint coincident P1 L21
  constraint midpoint P1 L8
  constraint perpendicular L17 L19
  constraint coincident L15.end L14
  constraint coincident L15.end L17
  constraint coincident L5.end L7
  constraint coincident L5.end L17
  constraint coincident L11.start L7
  constraint coincident L11.start L23
  constraint coincident L22.start L23
  constraint coincident L22.start L14
  constraint midpoint L6.end L28
  constraint horizontal L0
  constraint perpendicular L0 L32
  constraint parallel L0 L4
  constraint parallel L3 L32
  constraint coincident P0 L18
  constraint coincident P0 L24
  constraint midpoint P0 L6
  measures "d314" distance of L1.start L1.end
  measures "d315" distance of L17.start L1.start
  measures "d316" distance of L14.start L14.end
  measures "d317" distance of L14.start L5.start
  measures "d318" distance of L8.start L6.start
  measures "d319" distance of L9.start L10.end
  measures "d320" distance of L0.start L0.end
  measures "d321" distance of L4.start L0.end
sketch "MF3 2R 12P" plane through (0, 0, 0) normal (0, 1, 0) x (1, 0, 0) in component "Molex Micro Fit 3"
  line L0 (-0.85, -4.975) -> (0.85, -3.575) construction
  line L1 (-9.575, 3.575) -> (9.575, -3.575) construction
  line L2 (0.85, -4.975) -> (-0.85, -3.575) construction
  line L3 (-11.75, 1.875) -> (11.75, -1.875) construction
  line L4 (-9.575, 3.575) -> (-9.575, -3.575) construction
  line L5 (0.85, -3.575) -> (9.575, -3.575)
  line L6 (9.575, 3.575) -> (-9.575, -3.575) construction
  line L7 (-0.85, -3.575) -> (-9.575, -3.575)
  line L8 (9.575, 3.575) -> (-9.575, 3.575)
  line L9 (0, -3.575) -> (0, -4.975) construction
  line L10 (-9.575, -3.575) -> (-9.575, -1.875)
  line L11 (0, -4.975) -> (0, 3.575) construction
  line L12 (13.25, 4.8) -> (13.25, -6.2)
  line L13 (11.75, 1.875) -> (-11.75, -1.875) construction
  line L14 (0.85, -4.975) -> (-0.85, -4.975)
  line L15 (-13.25, -6.2) -> (-13.25, 4.8)
  line L16 (-13.25, 4.8) -> (13.25, 4.8)
  line L17 (9.575, 1.875) -> (9.575, 3.575)
  line L18 (-9.575, -1.875) -> (-11.75, -1.875)
  line L19 (9.575, 1.875) -> (11.75, 1.875)
  line L20 (9.575, -1.875) -> (11.75, -1.875)
  line L21 (9.575, -3.575) -> (9.575, 3.575) construction
  line L22 (0.85, -3.575) -> (0.85, -4.975)
  line L23 (-11.75, 1.875) -> (-11.75, -1.875)
  line L24 (11.75, -1.875) -> (11.75, 1.875)
  line L25 (-9.575, 1.875) -> (-9.575, 3.575)
  line L26 (-0.85, -4.975) -> (-0.85, -3.575)
  line L27 (-11.75, 1.875) -> (-9.575, 1.875)
  line L28 (-9.575, -3.575) -> (9.575, -3.575) construction
  line L29 (11.75, 1.875) -> (-11.75, 1.875) construction
  line L30 (9.575, -3.575) -> (9.575, -1.875)
  line L31 (-11.75, -1.875) -> (11.75, -1.875) construction
  line L32 (-0.85, -3.575) -> (0.85, -3.575) construction
  line L33 (13.25, -6.2) -> (-13.25, -6.2)
  line L34 (13.25, -6.2) -> (-13.25, 4.8) construction
  line L35 (-13.25, -6.2) -> (13.25, 4.8) construction
  point P0 (-1.5, 0)
  point P1 (0, -0.7)
  point P2 (0, -4.275)
  dimension "d322" = 19.15
  dimension "d323" = 7.15
  dimension "d324" = 23.5
  dimension "d325" = 3.75
  dimension "d326" = 1.4
  dimension "d327" = 1.7
  dimension "d328" = 26.5
  dimension "d329" = 11
  constraint horizontal L8
  constraint perpendicular L4 L8
  constraint parallel L8 L28
  constraint parallel L4 L21
  constraint coincident origin L6
  constraint coincident origin L1
  constraint horizontal L29
  constraint perpendicular L23 L29
  constraint parallel L29 L31
  constraint parallel L23 L24
  constraint coincident origin L13
  constraint coincident origin L3
  constraint midpoint L9.start L28
  constraint perpendicular L9 L28
  constraint horizontal L14
  constraint perpendicular L14 L26
  constraint parallel L14 L32
  constraint parallel L22 L26
  constraint coincident P2 L2
  constraint coincident P2 L0
  constraint midpoint P2 L9
  constraint perpendicular L4 L7
  constraint coincident L10.end L31
  constraint coincident L10.end L4
  constraint coincident L25.start L29
  constraint coincident L25.start L4
  constraint coincident L17.start L29
  constraint coincident L17.start L21
  constraint coincident L20.start L21
  constraint coincident L20.start L31
  constraint midpoint L11.end L8
  constraint horizontal L33
  constraint perpendicular L15 L33
  constraint parallel L16 L33
  constraint parallel L12 L15
  constraint coincident P1 L34
  constraint coincident P1 L35
  constraint midpoint P1 L11
  measures "d322" distance of L4.end L1.end
  measures "d323" distance of L1.start L4.end
  measures "d324" distance of L13.end L3.end
  measures "d325" distance of L13.end L3.start
  measures "d326" distance of L9.start L9.end
  measures "d327" distance of L0.end L2.end
  measures "d328" distance of L15.start L12.end
  measures "d329" distance of L15.start L15.end
sketch "MF3 2R 16P" plane through (0, 0, 0) normal (0, 1, 0) x (1, 0, 0) in component "Molex Micro Fit 3"
  line L0 (14.75, 1.875) -> (-14.75, 1.875) construction
  line L1 (-14.75, 1.875) -> (-14.75, -1.875)
  line L2 (-14.75, -1.875) -> (14.75, -1.875) construction
  line L3 (14.75, -1.875) -> (14.75, 1.875)
  line L4 (14.75, 1.875) -> (-14.75, -1.875) construction
  line L5 (-14.75, 1.875) -> (14.75, -1.875) construction
  line L6 (12.575, 3.575) -> (-12.575, 3.575)
  line L7 (-12.575, 3.575) -> (-12.575, -3.575) construction
  line L8 (-12.575, -3.575) -> (12.575, -3.575) construction
  line L9 (12.575, -3.575) -> (12.575, 3.575) construction
  line L10 (12.575, 3.575) -> (-12.575, -3.575) construction
  line L11 (-12.575, 3.575) -> (12.575, -3.575) construction
  line L12 (0, -3.575) -> (0, -4.975) construction
  line L13 (0.85, -3.575) -> (-0.85, -3.575) construction
  line L14 (-0.85, -3.575) -> (-0.85, -4.975)
  line L15 (-0.85, -4.975) -> (0.85, -4.975)
  line L16 (0.85, -4.975) -> (0.85, -3.575)
  line L17 (0.85, -3.575) -> (-0.85, -4.975) construction
  line L18 (-0.85, -3.575) -> (0.85, -4.975) construction
  line L19 (14.75, -1.875) -> (12.575, -1.875)
  line L20 (12.575, -1.875) -> (12.575, -3.575)
  line L21 (12.575, -3.575) -> (0.85, -3.575)
  line L22 (-0.85, -3.575) -> (-12.575, -3.575)
  line L23 (-12.575, -3.575) -> (-12.575, -1.875)
  line L24 (-12.575, -1.875) -> (-14.75, -1.875)
  line L25 (-14.75, 1.875) -> (-12.575, 1.875)
  line L26 (-12.575, 1.875) -> (-12.575, 3.575)
  line L27 (14.75, 1.875) -> (12.575, 1.875)
  line L28 (12.575, 1.875) -> (12.575, 3.575)
  line L29 (0, -4.975) -> (0, 3.575) construction
  line L30 (16.25, 4.8) -> (-16.25, 4.8)
  line L31 (-16.25, 4.8) -> (-16.25, -6.2)
  line L32 (-16.25, -6.2) -> (16.25, -6.2)
  line L33 (16.25, -6.2) -> (16.25, 4.8)
  line L34 (16.25, 4.8) -> (-16.25, -6.2) construction
  line L35 (-16.25, 4.8) -> (16.25, -6.2) construction
  point P0 (0, -4.275)
  point P1 (0, -0.7)
  dimension "d194" = 29.5
  dimension "d195" = 3.75
  dimension "d196" = 25.15
  dimension "d197" = 7.15
  dimension "d198" = 1.4
  dimension "d199" = 1.7
  dimension "d200" = 11
  dimension "d201" = 32.5
  constraint horizontal L0
  constraint perpendicular L0 L1
  constraint parallel L0 L2
  constraint parallel L1 L3
  constraint coincident L4 origin
  constraint coincident L5 origin
  constraint horizontal L6
  constraint perpendicular L6 L7
  constraint parallel L6 L8
  constraint parallel L7 L9
  constraint coincident L10 origin
  constraint coincident L11 origin
  constraint midpoint L8 L12.start
  constraint perpendicular L8 L12
  constraint horizontal L13
  constraint perpendicular L13 L14
  constraint parallel L13 L15
  constraint parallel L14 L16
  constraint coincident L17 P0
  constraint coincident L18 P0
  constraint midpoint L12 P0
  constraint coincident L12.end L15
  constraint coincident L2 L19.end
  constraint coincident L9 L19.end
  constraint coincident L2 L23.end
  constraint coincident L7 L23.end
  constraint perpendicular L1 L24
  constraint coincident L0 L25.end
  constraint coincident L7 L25.end
  constraint coincident L0 L27.end
  constraint coincident L9 L27.end
  constraint midpoint L6 L29.end
  constraint horizontal L30
  constraint perpendicular L30 L31
  constraint parallel L30 L32
  constraint parallel L31 L33
  constraint coincident L34 P1
  constraint coincident L35 P1
  constraint midpoint L29 P1
  measures "d194" distance of L1.end L2.end
  measures "d195" distance of L0.end L1.end
  measures "d196" distance of L7.end L8.end
  measures "d197" distance of L6.end L7.end
  measures "d198" distance of L12.start L12.end
  measures "d199" distance of L14.end L15.end
  measures "d200" distance of L30.end L31.end
  measures "d201" distance of L31.end L32.end
sketch "80mm Fan Profile" plane through (0, 0, 0) normal (0, 1, 0) x (1, 0, 0) in component "Fans"
  circle A0 centre (0, 0) radius 39
  line L0 (35.75, 35.75) -> (-35.75, 35.75) construction
  line L1 (-35.75, 35.75) -> (-35.75, -35.75) construction
  line L2 (-35.75, -35.75) -> (35.75, -35.75) construction
  line L3 (35.75, -35.75) -> (35.75, 35.75) construction
  line L4 (35.75, 35.75) -> (-35.75, -35.75) construction
  line L5 (-35.75, 35.75) -> (35.75, -35.75) construction
  circle A1 centre (-35.75, -35.75) radius 1.8
  circle A2 centre (35.75, -35.75) radius 1.8
  circle A3 centre (35.75, 35.75) radius 1.8
  circle A4 centre (-35.75, 35.75) radius 1.8
  dimension "d215" = 78
  dimension "d216" = 71.5
  dimension "d217" = 71.5
  dimension "d218" = 3.6
  dimension "d219" = 3.6
  dimension "d220" = 3.6
  dimension "d222" = 3.6
  constraint coincident A0.centre origin
  constraint horizontal L0
  constraint perpendicular L0 L1
  constraint parallel L0 L2
  constraint parallel L1 L3
  constraint coincident L4 A0.centre
  constraint coincident L5 A0.centre
  constraint coincident L1.end L2.start
  constraint coincident L2.end L3.start
  constraint coincident L0.start L3.end
  constraint coincident L0.end L1.start
  measures "d215" diameter of A0
  measures "d216" distance of L1.end L2.end
  measures "d217" distance of L0.end L1.end
  measures "d218" diameter of A1
  measures "d219" diameter of A2
  measures "d220" diameter of A3
  measures "d222" diameter of A4
sketch "60mm Fan Profile" plane through (0, 0, 0) normal (0, 1, 0) x (1, 0, 0) in component "Fans"
  circle A0 centre (0, 0) radius 29
  line L0 (25, 25) -> (-25, 25) construction
  line L1 (-25, 25) -> (-25, -25) construction
  line L2 (-25, -25) -> (25, -25) construction
  line L3 (25, -25) -> (25, 25) construction
  line L4 (25, 25) -> (-25, -25) construction
  line L5 (-25, 25) -> (25, -25) construction
  circle A1 centre (-25, -25) radius 1.8
  circle A2 centre (25, -25) radius 1.8
  circle A3 centre (25, 25) radius 1.8
  circle A4 centre (-25, 25) radius 0
  circle A5 centre (-25, 25) radius 1.8
  dimension "d208" = 58
  dimension "d209" = 50
  dimension "d210" = 50
  dimension "d211" = 3.6
  dimension "d212" = 3.6
  dimension "d213" = 3.6
  dimension "d214" = 3.6
  constraint coincident A0.centre origin
  constraint horizontal L0
  constraint perpendicular L0 L1
  constraint parallel L0 L2
  constraint parallel L1 L3
  constraint coincident L4 A0.centre
  constraint coincident L5 A0.centre
  constraint coincident L1.end L2.start
  constraint coincident L2.end L3.start
  constraint coincident L0.start L3.end
  constraint coincident L0.end L1.start
  measures "d208" diameter of A0
  measures "d209" distance of L1.end L2.end
  measures "d210" distance of L0.end L1.end
  measures "d211" diameter of A1
  measures "d212" diameter of A2
  measures "d213" diameter of A3
  measures "d214" diameter of A5
sketch "USB A" plane through (0, 0, 0) normal (0, 1, 0) x (1, 0, 0) in component "USB"
  line L0 (-19.5, -7.5) -> (19.5, -7.5)
  line L1 (7.25, 6) -> (-7.25, -6) construction
  line L2 (-19.5, 7.5) -> (19.5, -7.5) construction
  line L3 (0, 0) -> (15.25, 0) construction
  line L4 (19.5, 7.5) -> (-19.5, -7.5) construction
  circle A0 centre (15.25, 0) radius 1.8
  line L5 (-7.25, -6) -> (7.25, -6)
  line L6 (-7.25, 6) -> (7.25, -6) construction
  line L7 (19.5, -7.5) -> (19.5, 7.5)
  line L8 (-19.5, 7.5) -> (-19.5, -7.5)
  line L9 (19.5, 7.5) -> (-19.5, 7.5)
  line L10 (0, 0) -> (0, -6) construction
  circle A1 centre (-15.25, 0) radius 1.8
  line L11 (7.25, 6) -> (-7.25, 6)
  line L12 (7.25, -6) -> (7.25, 6)
  line L13 (-7.25, 6) -> (-7.25, -6)
  dimension "d24" = 15.25
  dimension "d25" = 3.6
  dimension "d26" = 14.5
  dimension "d27" = 12
  dimension "d28" = 39
  dimension "d29" = 15
  constraint coincident L3.start L10.start
  constraint horizontal L3
  constraint coincident L3.end A0.centre
  constraint horizontal L11
  constraint perpendicular L11 L13
  constraint parallel L5 L11
  constraint parallel L12 L13
  constraint coincident L3.start L1
  constraint coincident L3.start L6
  constraint midpoint L10.end L5
  constraint symmetric A0 L10 A1
  constraint horizontal L9
  constraint perpendicular L8 L9
  constraint parallel L0 L9
  constraint parallel L7 L8
  constraint coincident L3.start L4
  constraint coincident L3.start L2
  measures "d24" distance of L3.end L3.start
  measures "d25" diameter of A0
  measures "d26" distance of L1.end L5.end
  measures "d27" distance of L1.end L6.start
  measures "d28" distance of L0.end L0.start
  measures "d29" distance of L0.start L2.start
sketch "USB-C" plane through (0, 0, 0) normal (0, 1, 0) x (1, 0, 0) in component "USB"
  line L0 (0, -2.5) -> (3.5, -2.5)
  arc A0 (3.5, -2.5) -> (4.5, -1.5) centre (3.5, -1.5) ccw
  line L1 (4.5, 0) -> (4.5, -1.5)
  arc A1 (4.5, 1.5) -> (3.5, 2.5) centre (3.5, 1.5) ccw
  line L2 (0, 2.5) -> (3.5, 2.5)
  line L3 (4.5, 0) -> (4.5, 1.5)
  arc A2 (-3.5, 2.5) -> (-4.5, 1.5) centre (-3.5, 1.5) ccw
  line L4 (-4.5, 0) -> (-4.5, 1.5)
  line L5 (0, 2.5) -> (-3.5, 2.5)
  arc A3 (-4.5, -1.5) -> (-3.5, -2.5) centre (-3.5, -1.5) ccw
  line L6 (-4.5, 0) -> (-4.5, -1.5)
  line L7 (0, -2.5) -> (-3.5, -2.5)
  circle A4 centre (-8.375, 0) radius 1.75
  circle A5 centre (8.375, 0) radius 1.75
  line L8 (12.5, 6) -> (-12.5, 6)
  line L9 (-12.5, 6) -> (-12.5, -6)
  line L10 (-12.5, -6) -> (12.5, -6)
  line L11 (12.5, -6) -> (12.5, 6)
  line L12 (12.5, 6) -> (-12.5, -6) construction
  line L13 (-12.5, 6) -> (12.5, -6) construction
  dimension "d297" = 25
  dimension "d298" = 12
  constraint horizontal L8
  constraint perpendicular L8 L9
  constraint parallel L8 L10
  constraint parallel L9 L11
  constraint coincident L12 origin
  constraint coincident L13 origin
  measures "d297" distance of L9.end L10.end
  measures "d298" distance of L8.end L9.end
sketch "JST SM 4P" plane through (0, 0, 0) normal (0, 1, 0) x (1, 0, 0) in component "JST SM"
  line L0 (-9.1, -10.15) -> (9.1, -10.15)
  line L1 (9.1, -10.15) -> (9.1, -0.05)
  line L2 (9.1, -0.05) -> (-9.1, -0.05)
  line L3 (-9.1, -0.05) -> (-9.1, -10.15)
  line L4 (-7.5, -2.15) -> (-5.35, -2.15)
  line L5 (-7.5, -6.45) -> (-7.5, -2.15)
  line L6 (-5.35, -6.45) -> (-7.5, -6.45)
  line L7 (-5.35, -6.45) -> (-5.35, -6.95)
  line L8 (-5.35, -6.95) -> (-2.075, -6.95)
  line L9 (-2.075, -6.95) -> (-2.075, -8.55)
  line L10 (-2.075, -8.55) -> (2.075, -8.55)
  line L11 (2.075, -8.55) -> (2.075, -6.95)
  line L12 (2.075, -6.95) -> (5.35, -6.95)
  line L13 (5.35, -6.95) -> (5.35, -6.45)
  line L14 (7.5, -6.45) -> (5.35, -6.45)
  line L15 (7.5, -2.15) -> (7.5, -6.45)
  line L16 (5.35, -2.15) -> (7.5, -2.15)
  line L17 (5.35, -2.15) -> (5.35, -1.65)
  line L18 (-5.35, -1.65) -> (-5.35, -2.15)
  line L19 (5.35, -1.65) -> (-5.35, -1.65)
sketch "JST SM 5P" plane through (0, 0, 0) normal (0, 1, 0) x (1, 0, 0) in component "JST SM"
  line L0 (-10.35, -10.15) -> (10.35, -10.15)
  line L1 (10.35, -10.15) -> (10.35, -0.05)
  line L2 (10.35, -0.05) -> (-10.35, -0.05)
  line L3 (-10.35, -0.05) -> (-10.35, -10.15)
  line L4 (-8.75, -2.15) -> (-6.6, -2.15)
  line L5 (-8.75, -6.45) -> (-8.75, -2.15)
  line L6 (-6.6, -6.45) -> (-8.75, -6.45)
  line L7 (-6.6, -6.45) -> (-6.6, -6.95)
  line L8 (-6.6, -6.95) -> (-2.075, -6.95)
  line L9 (-2.075, -6.95) -> (-2.075, -8.55)
  line L10 (-2.075, -8.55) -> (2.075, -8.55)
  line L11 (2.075, -8.55) -> (2.075, -6.95)
  line L12 (2.075, -6.95) -> (6.6, -6.95)
  line L13 (6.6, -6.95) -> (6.6, -6.45)
  line L14 (8.75, -6.45) -> (6.6, -6.45)
  line L15 (8.75, -2.15) -> (8.75, -6.45)
  line L16 (6.6, -2.15) -> (8.75, -2.15)
  line L17 (6.6, -2.15) -> (6.6, -1.65)
  line L18 (-6.6, -1.65) -> (-6.6, -2.15)
  line L19 (6.6, -1.65) -> (-6.6, -1.65)
sketch "JST SM 3P" plane through (0, 0, 0) normal (0, 1, 0) x (1, 0, 0) in component "JST SM"
  line L0 (7.85, -0.25) -> (-7.85, -0.25)
  line L1 (-7.85, -0.25) -> (-7.85, -10.35)
  line L2 (-7.85, -10.35) -> (7.85, -10.35)
  line L3 (7.85, -10.35) -> (7.85, -0.25)
  line L4 (-6.25, -2.35) -> (-4.1, -2.35)
  line L5 (-6.25, -6.65) -> (-6.25, -2.35)
  line L6 (-4.1, -6.65) -> (-6.25, -6.65)
  line L7 (-4.1, -6.65) -> (-4.1, -7.15)
  line L8 (-4.1, -7.15) -> (-2.075, -7.15)
  line L9 (-2.075, -7.15) -> (-2.075, -8.75)
  line L10 (-2.075, -8.75) -> (2.075, -8.75)
  line L11 (2.075, -8.75) -> (2.075, -7.15)
  line L12 (2.075, -7.15) -> (4.1, -7.15)
  line L13 (4.1, -7.15) -> (4.1, -6.65)
  line L14 (6.25, -6.65) -> (4.1, -6.65)
  line L15 (6.25, -2.35) -> (6.25, -6.65)
  line L16 (4.1, -2.35) -> (6.25, -2.35)
  line L17 (4.1, -2.35) -> (4.1, -1.85)
  line L18 (-4.1, -1.85) -> (-4.1, -2.35)
  line L19 (4.1, -1.85) -> (-4.1, -1.85)
sketch "JST SM 2P" plane through (0, 0, 0) normal (0, 1, 0) x (1, 0, 0) in component "JST SM"
  line L0 (6.6, -0.25) -> (-6.6, -0.25)
  line L1 (-6.6, -0.25) -> (-6.6, -10.35)
  line L2 (-6.6, -10.35) -> (6.6, -10.35)
  line L3 (6.6, -10.35) -> (6.6, -0.25)
  line L4 (-5, -2.35) -> (-2.85, -2.35)
  line L5 (-5, -6.65) -> (-5, -2.35)
  line L6 (-2.85, -6.65) -> (-5, -6.65)
  line L7 (-2.85, -6.65) -> (-2.85, -7.15)
  line L8 (-2.85, -7.15) -> (-2.075, -7.15)
  line L9 (-2.075, -7.15) -> (-2.075, -8.75)
  line L10 (-2.075, -8.75) -> (2.075, -8.75)
  line L11 (2.075, -8.75) -> (2.075, -7.15)
  line L12 (2.075, -7.15) -> (2.85, -7.15)
  line L13 (2.85, -7.15) -> (2.85, -6.65)
  line L14 (5, -6.65) -> (2.85, -6.65)
  line L15 (5, -2.35) -> (5, -6.65)
  line L16 (2.85, -2.35) -> (5, -2.35)
  line L17 (2.85, -2.35) -> (2.85, -1.85)
  line L18 (-2.85, -1.85) -> (-2.85, -2.35)
  line L19 (2.85, -1.85) -> (-2.85, -1.85)